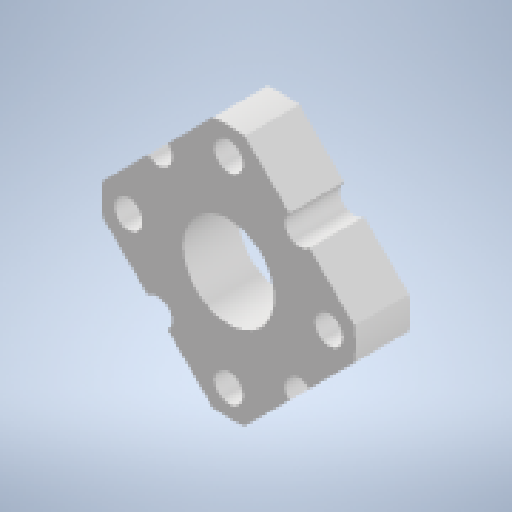
# Autodesk Inventor part: _arm_adt_64
Saved by Autodesk Inventor 2024.3 (Build 283343000, 343)
## iProperties
Created: 2024-09-06
Part Number: _arm_adt_64
Material: 일반
Document SubType Name: Modeling
Designer: gretc
Density: 1 g/cm^3
Appearance: 기본값
Author: gretc
Autodesk Inventor part; units mm, degrees
ref_plane "YZ Plane" through (0, 0, 0) normal (1, 0, 0) x (0, 1, 0)
ref_plane "XZ Plane" through (0, 0, 0) normal (0, 1, 0) x (-1, 0, 0)
ref_plane "XY Plane" through (0, 0, 0) normal (0, 0, 1) x (1, 0, 0)
sketch "스케치1" plane through (0, 0, 0) normal (0, 0, 1) x (1, 0, 0)
  circle A0 centre (-7.7782, -7.7782) radius 1.55 projected
  circle A1 centre (7.7782, -7.7782) radius 1.55 projected
  circle A2 centre (7.7782, 7.7782) radius 1.55 projected
  circle A3 centre (-7.7782, 7.7782) radius 1.55 projected
  circle A4 centre (0, 0) radius 5 projected
  circle A5 centre (0, 0) radius 13.9 projected
  circle A6 centre (0, 11) radius 1.55 projected
  circle A7 centre (11, 0) radius 1.55 projected
  circle A8 centre (0, -11) radius 1.55 projected
  circle A9 centre (-11, 0) radius 1.55 projected
  line L0 (0, -15.5563) -> (-15.5563, 0)
  line L1 (-15.5563, 0) -> (0, 15.5563)
  line L2 (0, 15.5563) -> (15.5563, 0)
  line L3 (15.5563, 0) -> (0, -15.5563)
  line L4 (0, -15.5563) -> (0, 15.5563) construction
  line L5 (-15.5563, 0) -> (15.5563, 0) construction
  circle A10 centre (0, 0) radius 1.5 projected
  circle A11 centre (0, 0) radius 2.5
  point P0 (0, 0)
  point P1 (1.7694, -13.7869)
  point P2 (6.6822, -8.8742)
  point P3 (8.8742, -6.6822)
  point P4 (13.7869, -1.7694)
  point P5 (13.7869, 1.7694)
  point P6 (8.8742, 6.6822)
  point P7 (6.6822, 8.8742)
  point P8 (1.7694, 13.7869)
  point P9 (-1.7694, 13.7869)
  point P10 (-6.6822, 8.8742)
  point P11 (-8.8742, 6.6822)
  point P12 (-13.7869, 1.7694)
  point P13 (-13.7869, -1.7694)
  point P14 (-8.8742, -6.6822)
  point P15 (-6.6822, -8.8742)
  point P16 (-1.7694, -13.7869)
  dimension "d0" = 5
  constraints: 12 end point, 2 midpoint, 2 parallel, 1 centre point, 1 coincident, 1 perpendicular
  measures "d0" diameter of A11
extrude "돌출1" add sketch "스케치1" along normal blind 6 contours A0 L0 A5 L1 A3 L2 A2 L3 A1
